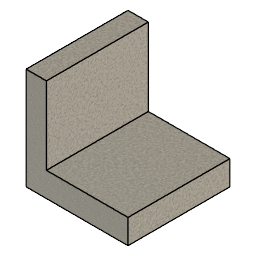
simulation nadec biju (Autodesk Fusion 360 design; units mm, degrees)
Autodesk Fusion 360 part; units mm, degrees
sketch "Sketch1" plane through (0, 0, 0) normal (0, 1, 0) x (1, 0, 0)
  line L0 (0, -50) -> (10, -50)
  line L1 (10, -50) -> (10, 0)
  line L2 (10, 0) -> (0, 0)
  line L3 (0, 0) -> (0, -50)
  line L4 (50, 0) -> (10, 0)
  line L5 (10, 0) -> (10, -12.0261)
  line L6 (10, -12.0261) -> (50, -12.0261)
  line L7 (50, -12.0261) -> (50, 0)
  constraint horizontal L0
  constraint vertical L1
  constraint horizontal L2
  constraint vertical L3
  constraint horizontal L4
  constraint vertical L5
  constraint horizontal L6
  constraint vertical L7
  constraint coincident L1 L5.end
extrude "Extrude1" add sketch "Sketch1" along normal mid plane 50
